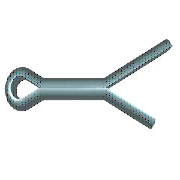
# Autodesk Inventor part: DIN EN ISO 1234 - 0,8x11
Saved by Autodesk Inventor 2024.4 (Build 284460000, 460)
## iProperties
Created: 2023-01-19
Part Number: DIN EN ISO 1234 - 0,8x11
Material: Stahl
Description: Splint
Document SubType Name: Modeling
Standard: DIN EN ISO 1234
Designer: windows-desktop
Standard Revision: 1998
Standards Organization: DIN
Language: de-DE
Size Designation: 0,8x11
Categories: <MemberInstance><Categories><Category DisplayName="Verbindungselemente" InternalName="e4da775c-781d-43d5-af7c-5136215cf5a6" Mnemonic="FSTN"><Category DisplayName="Stifte" InternalName="3b3d1810-ac9b-4ede-8c7f-cc6b956350b0" Mnemonic="PIN"><CategoryParameter DisplayName="Nenndurchmesser" InternalName="6cc331d7-8ea1-4fca-9c9a-55ec966217e5" Mnemonic="nomdia"/><CategoryParameter DisplayName="Nennlänge" InternalName="897bd938-6adf-4e3c-a2d4-0d7cae45eecd" Mnemonic="nomlen"/><Category DisplayName="Splinte" InternalName="4383ab9c-662d-4701-a95a-d5834a9f0a34" Mnemonic="SPLTPIN"><CategoryParameter DisplayName="Bolzendurchmesser" InternalName="761c08f3-f58b-48c9-8a5c-1931069602db" Mnemonic="bltdia"/></Category></Category></Category><Category DisplayName="Datentyp" InternalName="23b78d0f-2648-40c6-8793-ca6db495c9e8" Mnemonic="DATATYPE"><CategoryParameter DisplayName="Anzeigename" InternalName="05415f3d-3907-474b-a020-eb9d644f4cf3" Mnemonic="DISPLAYNAME"/><CategoryParameter DisplayName="Norm" InternalName="0c0a119c-1e12-4c84-803f-101930972f5e" Mnemonic="STANDARD"/><CategoryParameter DisplayName="Beschreibung" InternalName="13903e3d-64b1-4950-80da-f627842ea37f" Mnemonic="DESCRIPTION"/><CategoryParameter DisplayName="Bezeichnung" InternalName="2675968c-4ce5-49e0-a4f5-552d29089031" Mnemonic="DESIGNATION"/><CategoryParameter DisplayName="Standardzeile" InternalName="2af9ec52-faaa-4026-b378-f9fa4afca842" Mnemonic="DEFAULTROW"/><CategoryParameter DisplayName="Ordnername" InternalName="3f06958e-8713-4116-9be7-ed6184ecc97b" Mnemonic="FOLDERNAME"/><CategoryParameter DisplayName="Revisionsanleitung" InternalName="45a75005-10b1-4dfc-8d6d-dfe629f0b93c" Mnemonic="REVISIONGUID"/><CategoryParameter DisplayName="Dateiname" InternalName="8b46a4cc-9585-4fed-90c3-899f57e09a73" Mnemonic="FILENAME"/><CategoryParameter DisplayName="Normungsorganisation" InternalName="8f5914e1-4693-403f-8ab5-d37768198c9d" Mnemonic="STDSORG"/><CategoryParameter DisplayName="Gruppenversion" InternalName="914462f6-6e19-4b14-ba84-155b9680b1d0" Mnemonic="FAMILYREVISION"/><CategoryParameter DisplayName="Normrevision" InternalName="91d5a463-65c2-4fde-b823-3b7fea5e8e17" Mnemonic="STANDARDREVISION"/><CategoryParameter DisplayName="Variantenrevision" InternalName="a65d44b9-392f-4f4f-857b-e4b3d54996fe" Mnemonic="MEMBERREVISION"/><CategoryParameter DisplayName="ClipFormat" InternalName="bc51e27b-3422-4e78-93ef-cec197ddf230" Mnemonic="CLIPFORMAT"/><CategoryParameter DisplayName="Hersteller" InternalName="cd6c7a72-a28a-4e50-99a9-2c7f4e13e5ad" Mnemonic="MANUFACTURER"/><CategoryParameter DisplayName="InternerName" InternalName="cf1d0246-76d9-4b4a-8305-fa0409afb5c1" Mnemonic="INTERNALNAME"/><CategoryParameter DisplayName="IstMetrisch" InternalName="e2385c5b-1ea4-4823-96a8-8de651266ec3" Mnemonic="ISMETRIC"/><Category DisplayName="Bauteil" InternalName="c0e0b642-3bcb-4cc8-9e80-f96d35c4afa4" Mnemonic="PART"><CategoryParameter DisplayName="Bauteilnummer" InternalName="016b6077-bfbe-49bd-92c9-d8d59c39c941" Mnemonic="PARTNUMBER"/><CategoryParameter DisplayName="Bestandsnummer" InternalName="4dba7c1c-e26c-444e-836c-b08b433409a8" Mnemonic="STOCKNUMBER"/><CategoryParameter DisplayName="Materialschlüssel" InternalName="5c9a8adb-dd2b-4535-b97f-0a94a95fe41f" Mnemonic="MATERIALKEY"/><CategoryParameter DisplayName="Material" InternalName="818a152a-d3c3-49ca-80ee-df7d91421b8e" Mnemonic="MATERIAL"/></Category></Category><Category DisplayName="Abwärtskompatibilitätszuordnung DA" InternalName="924fff40-ddd0-4eff-ad42-30e3774ef79e" Mnemonic="LEGACYMAPDA"><CategoryParameter DisplayName="DA-Cookie" InternalName="316934ee-8fe1-4c7a-9c36-f2d79e1add1a" Mnemonic="DACOOKIE"/></Category></Categories><FamilyTemplate Id="I1234"><FamilyTemplateParameters><FamilyTemplateParameter ObjectType="kUserParameterObject" ValueType="xs:double" Id="1" ObjectReferenceKey="Diam"/><FamilyTemplateParameter ObjectType="kUserParameterObject" ValueType="xs:double" Id="2" ObjectReferenceKey="b"/><FamilyTemplateParameter ObjectType="kUserParameterObject" ValueType="xs:double" Id="3" ObjectReferenceKey="ParC"/><FamilyTemplateParameter ObjectType="kUserParameterObject" ValueType="xs:double" Id="4" ObjectReferenceKey="v"/><FamilyTemplateParameter ObjectType="kUserParameterObject" ValueType="xs:double" Id="5" ObjectReferenceKey="prf_lf"/><FamilyTemplateParameter ObjectType="kPropertyObject" ValueType="xs:string" Id="100" ObjectReferenceKey="{32853F0F-3444-11d1-9E93-0060B03C1CA6}" SubObjectId="52"/><FamilyTemplateParameter ObjectType="kPropertyObject" ValueType="xs:string" Id="105" ObjectReferenceKey="{32853F0F-3444-11d1-9E93-0060B03C1CA6}" SubObjectId="5"/><FamilyTemplateParameter ObjectType="kPartComponentDefinitionObject" ValueType="xs:string" Id="110" SubObjectId="Material"/></FamilyTemplateParameters></FamilyTemplate><CategoryParameterMap><ParamToTemplateMap><ParamToTemplate CategoryParameter="//CategoryParameter[@InternalName='05415f3d-3907-474b-a020-eb9d644f4cf3']" ConstantValue="DIN EN ISO 1234"/><ParamToTemplate CategoryParameter="//CategoryParameter[@InternalName='cf1d0246-76d9-4b4a-8305-fa0409afb5c1']" ConstantValue="67C42278-F2D5-4625-986D-4FA8993154BA"/><ParamToTemplate CategoryParameter="//CategoryParameter[@InternalName='3f06958e-8713-4116-9be7-ed6184ecc97b']" ConstantValue="DIN EN ISO 1234"/><ParamToTemplate CategoryParameter="//CategoryParameter[@InternalName='914462f6-6e19-4b14-ba84-155b9680b1d0']" ConstantValue="10"/><ParamToTemplate CategoryParameter="//CategoryParameter[@InternalName='bc51e27b-3422-4e78-93ef-cec197ddf230']" ConstantValue="CF_INVENTOR.STDPARTS"/><ParamToTemplate CategoryParameter="//CategoryParameter[@InternalName='e2385c5b-1ea4-4823-96a8-8de651266ec3']" ConstantValue="true"/><ParamToTemplate CategoryParameter="//CategoryParameter[@InternalName='13903e3d-64b1-4950-80da-f627842ea37f']" ConstantValue="Split Pin"/><ParamToTemplate CategoryParameter="//CategoryParameter[@InternalName='8f5914e1-4693-403f-8ab5-d37768198c9d']" ConstantValue="DIN"/><ParamToTemplate CategoryParameter="//CategoryParameter[@InternalName='0c0a119c-1e12-4c84-803f-101930972f5e']" ConstantValue="DIN EN ISO 1234"/><ParamToTemplate CategoryParameter="//CategoryParameter[@InternalName='cd6c7a72-a28a-4e50-99a9-2c7f4e13e5ad']" TemplateParameter="104"/><ParamToTemplate CategoryParameter="//CategoryParameter[@InternalName='91d5a463-65c2-4fde-b823-3b7fea5e8e17']" ConstantValue="1998"/><ParamToTemplate CategoryParameter="//CategoryParameter[@InternalName='45a75005-10b1-4dfc-8d6d-dfe629f0b93c']" ConstantValue="d636b13d-daf7-487b-ba8c-6da00f38c3ff"/><ParamToTemplate CategoryParameter="//CategoryParameter[@InternalName='2af9ec52-faaa-4026-b378-f9fa4afca842']" ConstantValue="10"/><ParamToTemplate CategoryParameter="//CategoryParameter[@InternalName='8b46a4cc-9585-4fed-90c3-899f57e09a73']" ConstantValue="DIN EN ISO 1234 - 0,8x11 x 8 x 2,50"/><ParamToTemplate CategoryParameter="//CategoryParameter[@InternalName='a65d44b9-392f-4f4f-857b-e4b3d54996fe']" ConstantValue="B3FF5C55-8164-45A0-AE64-8DB32959911B"/><ParamToTemplate CategoryParameter="//CategoryParameter[@InternalName='6cc331d7-8ea1-4fca-9c9a-55ec966217e5']" ConstantValue="2,50"/><ParamToTemplate CategoryParameter="//CategoryParameter[@InternalName='897bd938-6adf-4e3c-a2d4-0d7cae45eecd']" ConstantValue="11"/><ParamToTemplate CategoryParameter="//CategoryParameter[@InternalName='316934ee-8fe1-4c7a-9c36-f2d79e1add1a']" ConstantValue="*DIN~I1234~0.8x11~0.8~11~2.5*"/><ParamToTemplate CategoryParameter="//CategoryParameter[@InternalName='2675968c-4ce5-49e0-a4f5-552d29089031']" TemplateParameter="100"/><ParamToTemplate CategoryParameter="//CategoryParameter[@InternalName='818a152a-d3c3-49ca-80ee-df7d91421b8e']" TemplateParameter="110"/><ParamToTemplate CategoryParameter="//CategoryParameter[@InternalName='016b6077-bfbe-49bd-92c9-d8d59c39c941']" TemplateParameter="105"/></ParamToTemplateMap></CategoryParameterMap></MemberInstance>
Mass: 0.057907 g
Surface Area: 0.617644 cm^2
Volume: 0.00737668 cm^3
Density: 7.85 g/cm^3
Sheet Metal Rule: Standard
Appearance: Platte
IsCustomPart: 0
Author: windows-desktop
Autodesk Inventor part; units mm, degrees
sketch "Skizze1" plane through (0, 0, 0) normal (0, 0, 1) x (1, 0, 0)
  line L0 (4, 0.4) -> (-4, 0.4)
  line L1 (-4, 0.4) -> (-5.57377, 0.688525)
  arc A0 (-5.57377, 0.688525) -> (-5.57377, -0.688525) centre (-5.7, 0) ccw
  line L2 (-5.57377, -0.688525) -> (-4, -0.4)
  line L3 (-4, -0.4) -> (4, -0.4)
  line L4 (4, -0.01) -> (-4.035455, -0.01)
  line L5 (-4.035455, -0.01) -> (-5.644098, -0.304918)
  arc A1 (-5.644098, 0.304918) -> (-5.644098, -0.304918) centre (-5.7, 0) ccw
  line L6 (-5.644098, 0.304918) -> (-4.035455, 0.01)
  line L7 (-4.035455, 0.01) -> (4, 0.01)
  arc A2 (4, 0.4) -> (6.6205, 1.79528) centre (4, 3.558443) ccw
  arc A3 (4, 0.01) -> (6.944076, 1.577568) centre (4, 3.558443) ccw
  arc A4 (8.471436, -2.574903) -> (4, -0.01) centre (4, -5.190014) ccw
  arc A5 (8.134784, -2.771793) -> (4, -0.4) centre (4, -5.190014) ccw
  line L8 (6.6205, 1.79528) -> (7, 2.01)
  line L9 (7, 2.01) -> (6.944076, 1.577568)
  line L10 (8.471436, -2.574903) -> (8.5, -3.01)
  line L11 (8.134784, -2.771793) -> (8.5, -3.01)
  line L12 (-49.8, 0) -> (53.8, 0)
  line L13 (4, 0.4) -> (4, 0.01) construction
  line L14 (4, -0.01) -> (4, -0.4) construction
  line L15 (-6.4, 0) -> (-6.4, 40.080229) construction
  line L16 (-5.57377, 0.688525) -> (-5.644098, 0.304918) construction
  line L17 (6.6205, 1.79528) -> (6.944076, 1.577568) construction
  line L18 (6.782288, 1.686424) -> (7, 2.01) construction
  line L19 (8.471436, -2.574903) -> (8.134784, -2.771793) construction
  line L20 (8.30311, -2.673348) -> (8.5, -3.01) construction
  line L21 (0, 30.80959) -> (0, -39.73949)
  line L22 (-4, -0.4) -> (4, 0.4) construction
  point P0 (0, 0)
  dimension "d1" = 3
  dimension "d2" = 2
  dimension "d10" = 1.4
  dimension "d11" = 0.8
  dimension "d12" = 0.39
  dimension "d13" = 2.4
  dimension "d15" = 8
  dimension "d16" = 3
  dimension "d17" = 4.5
  dimension "d26" = 0.39
  constraints: 42 end point, 13 point on circle, 9 tangent, 6 centre point, 6 parallel, 5 equal length, 5 vertical alignment, 3 concentric, 3 midpoint, 3 perpendicular, 2 point on line, 1 collinear, 1 horizontal, 1 other
  measures "d1" horizontal distance of L8.end A2.centre
  measures "d2" vertical distance of L8.end L7.end
  measures "d10" diameter of A0
  measures "d11" distance between parallel lines of L3 L0
  measures "d12" distance of L4.start L3.end
  measures "d13" distance from line of L2.end L15
  measures "d15" distance of L3.end L2.end
  measures "d16" distance from line of L4 L10.end
  measures "d17" horizontal distance of L10.end A4.centre
  measures "d26" distance of L1.end L6.start
extrude "Extrusion1" add sketch "Skizze1" along normal mid plane 0.8 contours A2 L8 L9 A3 L7 L21 L0 | L21 L7 L6 A1 L12 A0 L1 L0 | L12 A1 L5 L4 L21 L3 L2 A0 | L4 A4 L10 L11 A5 L3 L21
fillet "Rundung1" radius 0.39 16 edges at (0, 0.4, 0.4) (5.4844, 0.7706, 0.4) (0, -0.4, 0.4) (6.3834, -1.035, 0.4) (-4.7869, -0.5443, 0.4) (-6.4, 0, 0.4) (-4.7869, 0.5443, 0.4) (-6.4, 0, -0.4) (-4.7869, -0.5443, -0.4) (-4.7869, 0.5443, -0.4) (0, 0.4, -0.4) (5.4844, 0.7706, -0.4) (0, -0.4, -0.4) (6.3834, -1.035, -0.4) (-4, 0.4, 0) (-4, -0.4, 0)
ref_plane "MSC_PF1" through (0, 0, 0) normal (1, 0, 0) x (0, 1, 0)
ref_plane "MSC_PT1" through (2.51607, -0.01, -0.4) normal (0, 0, -1) x (-1, 0, 0)
ref_plane "IDS_WORKPLANE{1}" through (-3.964545, -0.4, 0.01) normal (1, 0, 0) x (0, 1, 0)
equation "\"d1\" = v"
equation "\"d2\" = 0.666667 * d1"
equation "\"d10\" = ParC"
equation "\"d11\" = Diam"
equation "\"d13\" = b"
equation "\"d15\" = prf_lf"
equation "\"d16\" = 1.5 * d2"
equation "\"d17\" = 1.5 * d1"
equation "\"d26\" = d12"
equation "\"d18\" = Diam"
equation "\"d20\" = d12"
equation "\"msp_BendRadius\" = msp_Thickness"
equation "\"msp_BendReliefWidth\" = msp_Thickness"
equation "\"msp_BendReliefDepth\" = 0.5 * msp_Thickness"
equation "\"msp_CornerReliefSize\" = 4 * msp_Thickness"
equation "\"msp_MinimumRemnant\" = 2 * msp_Thickness"
equation "\"msp_TransitionRadius\" = msp_BendRadius"
equation "\"b\" = 2.4"
equation "\"ParC\" = 1.4"
equation "\"Diam\" = 0.8"
equation "\"v\" = 3"
equation "\"prf_lf\" = 8"
equation "\"JacobiRadiusSize\" = msp_Thickness"
equation "\"GapSize\" = msp_Thickness"
equation "\"msp_Thickness\" = 0.5"
body "Solid1"
